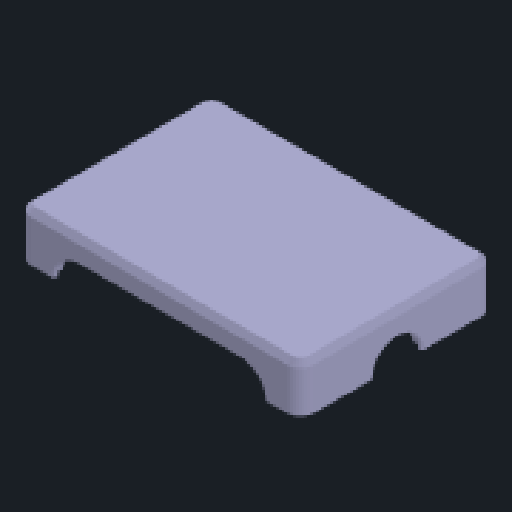
# Autodesk Inventor part: case2
Saved by Autodesk Inventor 2026.2 (Build 302298000, 298)
## iProperties
Created: 2025-10-05
Part Number: case2
Material: Generic
Document SubType Name: Modeling
Designer: micyg
Density: 1 g/cm^3
Appearance: Default
Sheet Metal Rule: Default
Author: micyg
## iProperties of the stored document case2_3DPrint.ipt
Created: 2025-10-05
Part Number: case2_3DPrint
Material: Generic
Document SubType Name: Modeling
Designer: micyg
Density: 1 g/cm^3
Appearance: Default
Author: micyg
Autodesk Inventor part; units mm, degrees
ref_plane "YZ Plane" through (0, 0, 0) normal (1, 0, 0) x (0, 1, 0)
ref_plane "XZ Plane" through (0, 0, 0) normal (0, 1, 0) x (-1, 0, 0)
ref_plane "XY Plane" through (0, 0, 0) normal (0, 0, 1) x (1, 0, 0)
sketch "Sketch1" plane through (0, 0, 0) normal (0, 1, 0) x (-1, 0, 0)
  line L0 (0, 0) -> (105, 0)
  line L1 (105, 0) -> (105, -72)
  line L2 (105, -72) -> (0, -72)
  line L3 (0, -72) -> (0, 0)
  dimension "d0" = 105
  dimension "d1" = 72
  constraints: 8 end point, 2 parallel, 1 horizontal, 1 perpendicular
  measures "d0" distance of L1.end L2.end
  measures "d1" distance of L0.end L1.end
extrude "Extrusion1" add sketch "Sketch1" along normal blind 17.5
fillet "Fillet1" radius 5 4 edges at (-105, 8.75, 0) (0, 8.75, 0) (-105, 8.75, -72) (0, 8.75, -72)
chamfer "Chamfer1" distance 2 angle 45 8 edges at (-52.5, 17.5, 0) (-1.4645, 17.5, -1.4645) (0, 17.5, -36) (-1.4645, 17.5, -70.5355) (-52.5, 17.5, -72) (-103.5355, 17.5, -70.5355) (-105, 17.5, -36) (-103.5355, 17.5, -1.4645)
shell "Shell2" thickness 3 removed faces 1 at (-36.6667, 0, -24)
ref_plane "Work Plane2" through (-52.5, 0, 0) normal (1, 0, 0) x (0, 1, 0)
ref_plane "Work Plane3" through (0, 0, -36) normal (0, 0, -1) x (-1, 0, 0)
ref_plane "Work Plane4" through (0, 1.915, 0) normal (0, -1, 0) x (1, 0, 0)
sketch "Sketch19" plane through (-52.5, 0, 0) normal (1, 0, 0) x (0, 1, 0)
  line L0 (0, -3) -> (14.2574, -3) projected
  line L1 (14.2574, -3) -> (0, -3) projected
  line L2 (14.5, -5.7) -> (8.5, -5.7)
  line L3 (7.5, -5.7) -> (8.5, -6.7) construction
  line L4 (8.5, -6.7) -> (8.5, -5.7)
  line L5 (8.5, -5.7) -> (7.5, -5.7) construction
  line L6 (8.5, -6.7) -> (14.5, -12.7)
  line L7 (0, -67) -> (0, -72) projected
  line L8 (0, -5) -> (0, -67) projected
  line L9 (0, 0) -> (0, -5) projected
  line L10 (0, -5) -> (0, 0) projected
  line L11 (0, -67) -> (0, -5) projected
  line L12 (0, -72) -> (0, -67) projected
  line L13 (14.5, -3.2426) -> (14.5, -5) projected
  line L14 (14.5, -5) -> (14.5, -67) projected
  line L15 (14.5, -67) -> (14.5, -68.7574) projected
  line L16 (14.5, -68.7574) -> (14.5, -67) projected
  line L17 (14.5, -67) -> (14.5, -5) projected
  line L18 (14.5, -5) -> (14.5, -3.2426) projected
  dimension "d104" = 2.7
  dimension "d105" = 1
  dimension "d157" = 45
  dimension "d179" = 6
  constraints: 10 end point, 2 perpendicular, 2 point on line, 1 collinear
  measures "d104" distance between parallel lines of L0 L2
  measures "d105" distance from line of L3.end L2
  measures "d157" angle of L17 L6
  measures "d179" distance between parallel lines of L17 L4
extrude "Extrusion15" add sketch "Sketch19" against normal up to surface (49.5 mm away)
mirror "Mirror9" about plane through (-52.5, 0, 0) normal (1, 0, 0) of "Extrusion15"
mirror "Mirror10" about plane through (0, 0, -36) normal (0, 0, -1) of "Extrusion15", "Mirror9"
sketch "Sketch9" plane through (0, 1.915, 0) normal (0, -1, 0) x (1, 0, 0)
  arc A0 (-5, -72) -> (0, -67) centre (-5, -67) ccw projected
  line L0 (0, -5) -> (0, -67) projected
  arc A1 (0, -5) -> (-5, 0) centre (-5, -5) ccw projected
  line L1 (-100, 0) -> (-5, 0) projected
  arc A2 (-100, 0) -> (-105, -5) centre (-100, -5) ccw projected
  line L2 (-105, -67) -> (-105, -5) projected
  arc A3 (-105, -67) -> (-100, -72) centre (-100, -67) ccw projected
  line L3 (-5, -72) -> (-100, -72) projected
  line L4 (-96.5, -8.5) -> (-8.5, -8.5) construction
  line L5 (-8.5, -8.5) -> (-8.5, -63.5) construction
  line L6 (-8.5, -63.5) -> (-96.5, -63.5) construction
  line L7 (-96.5, -63.5) -> (-96.5, -8.5) construction
  circle A4 centre (-96.5, -8.5) radius 1.5
  circle A5 centre (-8.5, -8.5) radius 1.5
  circle A6 centre (-96.5, -63.5) radius 1.5
  circle A7 centre (-8.5, -63.5) radius 1.5
  line L8 (-52.5, -8.5) -> (-52.5, -63.5) construction
  line L9 (-101.5, -3.5) -> (-3.5, -3.5) construction
  line L10 (-3.5, -3.5) -> (-3.5, -68.5) construction
  line L11 (-3.5, -68.5) -> (-101.5, -68.5) construction
  line L12 (-101.5, -68.5) -> (-101.5, -3.5) construction
  line L13 (-101.5, -36) -> (-3.5, -36) construction
  line L14 (-52.5, 0) -> (-52.5, -72) construction
  line L15 (-105, -36) -> (0, -36) construction
  line L16 (-93, -3) -> (-93, -8.5)
  line L17 (-102.2, -12) -> (-102.2, -5)
  arc A8 (-96.5, -12) -> (-93, -8.5) centre (-96.5, -8.5) ccw
  line L18 (-96.5, -12) -> (-102.2, -12)
  line L19 (-100.2, -3) -> (-93, -3)
  line L20 (-93, -69) -> (-93, -63.5)
  arc A9 (-93, -63.5) -> (-96.5, -60) centre (-96.5, -63.5) ccw
  line L21 (-96.5, -60) -> (-102.2, -60)
  arc A10 (-12, -8.5) -> (-8.5, -12) centre (-8.5, -8.5) ccw
  line L22 (-3, -12) -> (-3, -5)
  line L23 (-12, -3) -> (-12, -8.5)
  line L24 (-8.5, -12) -> (-3, -12)
  line L25 (-5, -3) -> (-12, -3)
  arc A11 (-8.5, -60) -> (-12, -63.5) centre (-8.5, -63.5) ccw
  line L26 (-12, -69) -> (-12, -63.5)
  line L27 (-8.5, -60) -> (-3, -60)
  line L28 (-93, -3) -> (-95, -3)
  line L29 (-95, -3) -> (-95, -5.7)
  line L30 (-95, -5.7) -> (-93, -5.7)
  line L31 (-93, -5.7) -> (-93, -3)
  line L32 (-12, -3) -> (-10, -3)
  line L33 (-10, -3) -> (-10, -5.7)
  line L34 (-10, -5.7) -> (-12, -5.7)
  line L35 (-12, -5.7) -> (-12, -3)
  line L36 (-95, -69) -> (-95, -66.3)
  line L37 (-95, -66.3) -> (-93, -66.3)
  line L38 (-10, -69) -> (-10, -66.3)
  line L39 (-10, -66.3) -> (-12, -66.3)
  arc A12 (-3, -5) -> (-5, -3) centre (-5, -5) ccw projected
  line L40 (-5, -3) -> (-100, -3) projected
  line L41 (-3, -67) -> (-3, -5) projected
  arc A13 (0, -5) -> (-5, 0) centre (-5, -5) ccw projected
  line L42 (0, -5) -> (0, -67) projected
  line L43 (-100, 0) -> (-5, 0) projected
  arc A14 (-3, -5) -> (-5, -3) centre (-5, -5) ccw projected
  line L44 (-5, -3) -> (-100, -3) projected
  line L45 (-3, -67) -> (-3, -5) projected
  arc A15 (0, -5) -> (-5, 0) centre (-5, -5) ccw projected
  line L46 (0, -5) -> (0, -67) projected
  line L47 (-100, 0) -> (-5, 0) projected
  arc A16 (-5, -69) -> (-3, -67) centre (-5, -67) ccw projected
  line L48 (-5, -69) -> (-100, -69) projected
  arc A17 (-102, -67) -> (-100, -69) centre (-100, -67) ccw projected
  line L49 (-102, -67) -> (-102, -5) projected
  arc A18 (-100, -3) -> (-102, -5) centre (-100, -5) ccw projected
  line L50 (-100, -3) -> (-5, -3) projected
  arc A19 (-3, -5) -> (-5, -3) centre (-5, -5) ccw projected
  line L51 (-3, -5) -> (-3, -67) projected
  arc A20 (-5, -72) -> (0, -67) centre (-5, -67) ccw projected
  line L52 (0, -5) -> (0, -67) projected
  arc A21 (0, -5) -> (-5, 0) centre (-5, -5) ccw projected
  line L53 (-100, 0) -> (-5, 0) projected
  arc A22 (-100, 0) -> (-105, -5) centre (-100, -5) ccw projected
  line L54 (-105, -67) -> (-105, -5) projected
  arc A23 (-105, -67) -> (-100, -72) centre (-100, -67) ccw projected
  line L55 (-5, -72) -> (-100, -72) projected
  line L56 (-102, -6.7) -> (-102, -5.7) projected
  line L57 (-3, -6.7) -> (-102, -6.7) construction
  line L58 (-3, -5.7) -> (-3, -6.7) projected
  line L59 (-102, -5.7) -> (-3, -5.7) construction
  line L60 (-102, -66.3) -> (-102, -65.3) projected
  line L61 (-3, -66.3) -> (-102, -66.3) construction
  line L62 (-3, -65.3) -> (-3, -66.3) projected
  line L63 (-102, -65.3) -> (-3, -65.3) construction
  arc A24 (-5, -69) -> (-3, -67) centre (-5, -67) ccw projected
  arc A25 (-100, -3) -> (-102, -5) centre (-100, -5) ccw projected
  line L64 (-102, -5) -> (-102, -67) projected
  arc A26 (-102, -67) -> (-100, -69) centre (-100, -67) ccw projected
  line L65 (-100, -69) -> (-5, -69) projected
  arc A27 (-5, -72) -> (0, -67) centre (-5, -67) ccw projected
  line L66 (-5, -72) -> (-100, -72) projected
  arc A28 (-105, -67) -> (-100, -72) centre (-100, -67) ccw projected
  line L67 (-105, -67) -> (-105, -5) projected
  arc A29 (-100, 0) -> (-105, -5) centre (-100, -5) ccw projected
  line L68 (-102, -5) -> (-102, -67) projected
  line L69 (-105, -67) -> (-105, -5) projected
  arc A30 (-102, -67) -> (-100, -69) centre (-100, -67) ccw projected
  line L70 (-100, -69) -> (-5, -69) projected
  line L71 (-5, -72) -> (-100, -72) projected
  arc A31 (-105, -67) -> (-100, -72) centre (-100, -67) ccw projected
  arc A32 (-5, -69) -> (-3, -67) centre (-5, -67) ccw projected
  arc A33 (-100, -3) -> (-102, -5) centre (-100, -5) ccw projected
  arc A34 (-5, -72) -> (0, -67) centre (-5, -67) ccw projected
  arc A35 (-100, 0) -> (-105, -5) centre (-100, -5) ccw projected
  point P0 (-52.5, -36)
  point P1 (-12, -66.3)
  point P2 (-93, -66.3)
  point P3 (-10, -3)
  point P4 (-102, -60)
  point P5 (-95, -69)
  point P6 (-102, -12)
  point P7 (-10, -69)
  point P8 (-3, -67)
  dimension "d137" = 88
  dimension "d138" = 55
  dimension "d139" = 3
  dimension "d140" = 3
  dimension "d141" = 3
  dimension "d142" = 3
  dimension "d143" = 98
  dimension "d144" = 65
  dimension "d147" = 2
  dimension "d148" = 2
  dimension "d150" = 2
  dimension "d192" = 0.5
  constraints: 70 end point, 16 symmetric about line, 11 midpoint, 11 parallel, 8 centre point, 8 point on circle, 7 horizontal, 6 perpendicular, 5 coincident, 4 point on line, 4 tangent, 1 collinear, 6 other
  measures "d137" distance of L4.start L4.end
  measures "d138" distance of L6.end L4.start
  measures "d139" diameter of A4
  measures "d140" diameter of A7
  measures "d141" diameter of A5
  measures "d142" diameter of A6
  measures "d143" distance of L9.start L9.end
  measures "d144" distance of L12.start L9.start
  measures "d147" radial gap between concentric circles of A4 A8
  measures "d148" radial gap between concentric circles of A10 A5
  measures "d150" distance between parallel lines of L16 L29
  measures "d192" distance between parallel lines of L49 L12
extrude "Extrusion13" add sketch "Sketch9" against normal up to surface (12.585 mm away) contours L16 A8 L18 L49 A18 L19 L29 L30 | L34 L33 L25 A12 L22 L24 A10 L23 | L21 A9 L20 L37 L36 L48 A17 L49 | L41 A16 L48 L38 L39 L26 A11 L27
ref_plane "Work Plane6" through (0, 0, -24) normal (0, 0, -1) x (-1, 0, 0)
sketch "Sketch22" plane through (0, 0, -24) normal (0, 0, -1) x (-1, 0, 0)
  line L0 (3, 2.5) -> (15, 14.5)
  line L1 (90, 14.5) -> (102.1, 2.4)
  line L2 (3, 1.915) -> (3, 13.8) projected
  line L3 (3, 1.915) -> (3, 0) projected
  line L4 (3, 0) -> (3, 1.915) projected
  line L5 (3.2426, 14.5) -> (101.7574, 14.5) projected
  line L6 (101.7574, 14.5) -> (3.2426, 14.5) projected
  line L7 (102, 14.2574) -> (101.7574, 14.5) projected
  line L8 (101.7574, 14.5) -> (102, 14.2574) projected
  line L9 (102, 1.915) -> (102, 0) projected
  line L10 (102, 0) -> (102, 1.915) projected
  line L11 (52.5, -3.5) -> (52.5, 21) projected
  line L12 (102, 13.8) -> (102, 14.2574) projected
  line L13 (102, 14.2574) -> (102, 13.8) projected
  line L14 (3.2426, 14.5) -> (3, 14.2574) projected
  line L15 (3, 14.2574) -> (3.2426, 14.5) projected
  line L16 (3, 13.8) -> (3, 14.2574) projected
  line L17 (3, 14.2574) -> (3, 13.8) projected
  line L18 (10, 14.5) -> (95, 14.5) projected
  line L19 (95, 14.5) -> (10, 14.5) projected
  line L20 (10, 14.5) -> (95, 14.5) projected
  line L21 (95, 14.5) -> (10, 14.5) projected
  line L22 (102, 1.915) -> (102, 13.8) projected
  line L23 (102, 13.8) -> (102, 1.915) projected
  line L24 (3, 13.8) -> (3, 1.915) projected
  point P0 (3, 14.2574)
  point P1 (3.2426, 14.5)
  dimension "d184" = 12
  dimension "d185" = 45
  constraints: 4 end point, 3 point on line, 1 other
  measures "d184" distance from line of L5 L0.start
  measures "d185" angle of L6 L0
extrude "Extrusion18" add sketch "Sketch22" along normal mid plane 2 contours L2 L16 L14 L5 L0
mirror "Mirror12" about plane through (0, 0, -36) normal (0, 0, -1) of "Extrusion18"
sketch "Sketch26" plane through (0, 1.915, 0) normal (0, -1, 0) x (1, 0, 0)
  line L0 (-3, -60) -> (-3, -12) projected
  line L1 (0, -5) -> (0, -67) projected
  arc A0 (-5, -72) -> (0, -67) centre (-5, -67) ccw projected
  line L2 (-5, -72) -> (-100, -72) projected
  line L3 (-10, -5.7) -> (-10, -3) projected
  arc A1 (-3, -5) -> (-5, -3) centre (-5, -5) ccw projected
  arc A2 (0, -5) -> (-5, 0) centre (-5, -5) ccw projected
  line L4 (-100, 0) -> (-5, 0) projected
  line L5 (-10, -3) -> (-95, -3) projected
  line L6 (-12, -5.7) -> (-10, -5.7) projected
  line L7 (-12, -8.5) -> (-12, -5.7) projected
  arc A3 (-12, -8.5) -> (-8.5, -12) centre (-8.5, -8.5) ccw projected
  line L8 (-3, -12) -> (-8.5, -12) projected
  arc A4 (-100, 0) -> (-105, -5) centre (-100, -5) ccw projected
  line L9 (-105, -67) -> (-105, -5) projected
  arc A5 (-105, -67) -> (-100, -72) centre (-100, -67) ccw projected
  circle A6 centre (-96.5, -63.5) radius 1.5 projected
  circle A7 centre (-96.5, -8.5) radius 1.5 projected
  circle A8 centre (-8.5, -8.5) radius 1.5 projected
  circle A9 centre (-8.5, -63.5) radius 1.5 projected
  circle A10 centre (-8.5, -8.5) radius 1.5 projected
  circle A11 centre (-96.5, -63.5) radius 1.5 projected
  circle A12 centre (-8.5, -63.5) radius 1.5 projected
  circle A13 centre (-96.5, -8.5) radius 1.5 projected
  line L10 (-93, -5.7) -> (-93, -8.5) projected
  arc A14 (-96.5, -12) -> (-93, -8.5) centre (-96.5, -8.5) ccw projected
  line L11 (-96.5, -12) -> (-102, -12) projected
  line L12 (-102, -12) -> (-102, -5) projected
  line L13 (-100, -3) -> (-95, -3) projected
  line L14 (-95, -3) -> (-95, -5.7) projected
  line L15 (-95, -5.7) -> (-93, -5.7) projected
  line L16 (-102, -12) -> (-102, -60) projected
  line L17 (-102, -67) -> (-102, -60) projected
  line L18 (-95, -69) -> (-100, -69) projected
  line L19 (-95, -66.3) -> (-95, -69) projected
  line L20 (-93, -66.3) -> (-95, -66.3) projected
  line L21 (-93, -63.5) -> (-93, -66.3) projected
  arc A15 (-93, -63.5) -> (-96.5, -60) centre (-96.5, -63.5) ccw projected
  line L22 (-102, -60) -> (-96.5, -60) projected
  line L23 (-8.5, -60) -> (-3, -60) projected
  arc A16 (-8.5, -60) -> (-12, -63.5) centre (-8.5, -63.5) ccw projected
  line L24 (-12, -66.3) -> (-12, -63.5) projected
  line L25 (-10, -66.3) -> (-12, -66.3) projected
  line L26 (-10, -69) -> (-10, -66.3) projected
  line L27 (-95, -69) -> (-10, -69) projected
  line L28 (-10, -3) -> (-5, -3) projected
  line L29 (-3, -12) -> (-3, -5) projected
  line L30 (-3, -67) -> (-3, -60) projected
  line L31 (-5, -69) -> (-10, -69) projected
  arc A17 (-102, -67) -> (-100, -69) centre (-100, -67) ccw projected
  arc A18 (-5, -69) -> (-3, -67) centre (-5, -67) ccw projected
  arc A19 (-100, -3) -> (-102, -5) centre (-100, -5) ccw projected
  point P0 (0, 0)
extrude "Extrusion21" cut sketch "Sketch26" against normal up to surface (12.585 mm away) contours A6 | A7 | A8 | A9
sketch "Sketch30" plane through (0, 0, -5) normal (1, 0, 0) x (0, 0, -1)
  line L0 (0, 15.5) -> (62, 15.5) construction
  line L1 (0, 0) -> (0, 15.5) construction
  line L2 (0, 0) -> (62, 0) construction
  line L3 (62, 15.5) -> (62, 0) construction
  line L4 (31, 22.8) -> (31, -14.3) construction
  circle A0 centre (31, 0) radius 9
  point P0 (-5, 0)
  dimension "d160" = 18
  constraints: 1 centre point, 1 midpoint, 1 point on line
  measures "d160" diameter of A0
extrude "Extrusion22" cut sketch "Sketch30" against normal up to surface (3 mm away)
sketch "Sketch31" plane through (-5, 0, -72) normal (0, 0, -1) x (-1, 0, 0)
  line L0 (17.5, -9) -> (47.6, -9)
  arc A0 (17.5, 9) -> (17.5, -9) centre (17.5, 0) ccw
  line L1 (54.189, 9) -> (17.5, 9)
  line L2 (77.5, -9) -> (47.6, -9)
  arc A1 (77.5, -9) -> (77.5, 9) centre (77.5, 0) ccw
  line L3 (54.189, 9) -> (77.5, 9)
  line L4 (86.5, 9) -> (8.5, 9) construction
  line L5 (8.5, 9) -> (8.5, -9) construction
  line L6 (8.5, -9) -> (86.5, -9) construction
  line L7 (86.5, -9) -> (86.5, 9) construction
  line L8 (86.5, 9) -> (8.5, -9) construction
  line L9 (8.5, 9) -> (86.5, -9) construction
  line L10 (0, 15.5) -> (95, 15.5) projected
  line L11 (0, 0) -> (0, 15.5) projected
  line L12 (0, 0) -> (95, 0) projected
  line L13 (95, 15.5) -> (95, 0) projected
  line L14 (47.5, -14.3) -> (47.5, 22.8) projected
  point P0 (47.5, 0)
  point P1 (47.5, 0)
  point P2 (47.5, 0)
  point P3 (47.5, 0)
  dimension "d163" = 9
  dimension "d164" = 78
  constraints: 20 end point, 6 tangent, 5 midpoint, 4 point on circle, 3 collinear, 3 parallel, 3 point on line, 2 centre point, 1 coincident, 1 horizontal, 1 perpendicular, 1 other
  measures "d163" radius of A0
  measures "d164" distance between parallel lines of L5 L7
extrude "Extrusion23" cut sketch "Sketch31" against normal up to surface (3 mm away) contours A0 L12 L14 L0 | L14 L12 A1 L2 L0 | A0 L1 L14 L12 | L14 L1 L3 A1 L12
mirror "Mirror13" about plane through (0, 0, -36) normal (0, 0, -1) of "Extrusion23"
sketch "Sketch33" plane through (0, 0, 0) normal (0, -1, 0) x (1, 0, 0)
  line L0 (-91.5, -3) -> (-91.5, 0) projected
  line L1 (-100, 0) -> (-91.5, 0) projected
  arc A0 (-100, 0) -> (-105, -5) centre (-100, -5) ccw projected
  line L2 (-105, -67) -> (-105, -5) projected
  arc A1 (-105, -67) -> (-100, -72) centre (-100, -67) ccw projected
  line L3 (-91.5, -72) -> (-100, -72) projected
  line L4 (-91.5, -72) -> (-91.5, -69) projected
  line L5 (-91.5, -69) -> (-100, -69) projected
  arc A2 (-102, -67) -> (-100, -69) centre (-100, -67) ccw projected
  line L6 (-102, -67) -> (-102, -5) projected
  arc A3 (-100, -3) -> (-102, -5) centre (-100, -5) ccw projected
  line L7 (-100, -3) -> (-91.5, -3) projected
  line L8 (-13.5, 0) -> (-13.5, -3) projected
  line L9 (-13.5, -3) -> (-5, -3) projected
  arc A4 (-3, -5) -> (-5, -3) centre (-5, -5) ccw projected
  line L10 (-3, -5) -> (-3, -27) projected
  line L11 (-3, -27) -> (0, -27) projected
  line L12 (0, -5) -> (0, -27) projected
  arc A5 (0, -5) -> (-5, 0) centre (-5, -5) ccw projected
  line L13 (-13.5, 0) -> (-5, 0) projected
  line L14 (-13.5, -69) -> (-13.5, -72) projected
  line L15 (-5, -72) -> (-13.5, -72) projected
  arc A6 (-5, -72) -> (0, -67) centre (-5, -67) ccw projected
  line L16 (0, -45) -> (0, -67) projected
  line L17 (0, -45) -> (-3, -45) projected
  line L18 (-3, -45) -> (-3, -67) projected
  arc A7 (-5, -69) -> (-3, -67) centre (-5, -67) ccw projected
  line L19 (-5, -69) -> (-13.5, -69) projected
  arc A8 (-5, -70.6) -> (-1.4, -67) centre (-5, -67) ccw
  line L20 (-5, -70.6) -> (-13.5, -70.6)
  line L21 (-1.4, -45) -> (-1.4, -67)
  line L22 (-13.5, -1.4) -> (-5, -1.4)
  arc A9 (-1.4, -5) -> (-5, -1.4) centre (-5, -5) ccw
  line L23 (-1.4, -5) -> (-1.4, -27)
  line L24 (-103.6, -5) -> (-103.6, -67)
  arc A10 (-103.6, -67) -> (-100, -70.6) centre (-100, -67) ccw
  line L25 (-100, -70.6) -> (-91.5, -70.6)
  line L26 (-91.5, -1.4) -> (-100, -1.4)
  arc A11 (-100, -1.4) -> (-103.6, -5) centre (-100, -5) ccw
  line L27 (-13.5, 0) -> (-13.5, -3) projected
  line L28 (-91.5, -72) -> (-91.5, -69) projected
  line L29 (-91.5, -3) -> (-91.5, 0) projected
  line L30 (-3, -45) -> (-3, -27) projected
  line L31 (-1.4, -45) -> (-3, -45)
  line L32 (-3, -45) -> (-3, -27)
  line L33 (-3, -27) -> (-1.4, -27)
  line L34 (-1.4, -27) -> (-1.4, -45)
  line L35 (-91.5, -1.4) -> (-13.5, -1.4)
  line L36 (-13.5, -1.4) -> (-13.5, -3)
  line L37 (-13.5, -3) -> (-91.5, -3)
  line L38 (-91.5, -3) -> (-91.5, -1.4)
  line L39 (-5, -69) -> (-13.5, -69) projected
  line L40 (-13.5, -69) -> (-91.5, -69)
  line L41 (-91.5, -69) -> (-91.5, -70.6)
  line L42 (-91.5, -70.6) -> (-13.5, -70.6)
  line L43 (-13.5, -70.6) -> (-13.5, -69)
  point P0 (0, 0)
  point P1 (-13.5, -70.6)
  point P2 (-13.5, -1.4)
  point P3 (-91.5, -1.4)
  dimension "d174" = 1.4
  dimension "d175" = 1.4
  dimension "d176" = 1.4
  constraints: 38 end point, 8 point on circle, 6 parallel, 6 point on line, 4 centre point, 3 horizontal, 3 perpendicular, 2 tangent, 6 other
  measures "d174" distance between parallel lines of L1 L26
  measures "d175" distance between parallel lines of L13 L22
  measures "d176" distance between parallel lines of L16 L21
extrude "Extrusion25" cut sketch "Sketch33" against normal blind 1.6 contours L7 A3 L6 A2 L5 L4 L25 A10 L24 A11 L26 L0 | L0 L35 L8 L37 | L8 L22 A9 L23 L11 L10 A4 L9 | L11 L34 L17 L30 | L40 L14 L42 L4 | L17 L21 A8 L20 L14 L19 A7 L18
sketch "Sketch34" plane through (0, 0, -25) normal (0, 0, -1) x (-1, 0, 0)
  line L0 (3, 14.2574) -> (3, 2.5) projected
  line L1 (3.2426, 14.5) -> (3, 14.2574) projected
  line L2 (15, 14.5) -> (3.2426, 14.5) projected
  line L3 (15, 14.5) -> (3, 2.5) construction
  line L4 (15, 14.5) -> (3.2426, 14.5) projected
  line L5 (3.2426, 14.5) -> (15, 14.5) projected
  line L6 (101.7574, 14.5) -> (3.2426, 14.5) projected
  line L7 (3.2426, 14.5) -> (15, 14.5) projected
  line L8 (15, 14.5) -> (3.2426, 14.5) projected
  line L9 (3.2426, 14.5) -> (101.7574, 14.5) projected
  line L10 (5.6, 14.5) -> (5.6, 8.5)
  line L11 (5.6, 7.5) -> (6.6, 8.5) construction
  line L12 (5.6, 8.5) -> (6.6, 8.5)
  line L13 (6.6, 8.5) -> (12.6, 14.5)
  line L14 (5.6, 8.5) -> (5.6, 7.5) construction
  line L15 (93, 8.5) -> (12, 8.5) projected
  line L16 (12, 8.5) -> (93, 8.5) projected
  point P0 (0, 0)
  point P1 (12.6, 14.5)
  dimension "d180" = 1
  dimension "d181" = 45
  dimension "d183" = 2.6
  constraints: 10 end point, 2 collinear, 2 point on line, 2 vertical, 1 horizontal
  measures "d180" distance from line of L11.end L10
  measures "d181" angle of L9 L13
  measures "d183" distance between parallel lines of L0 L10
extrude "Extrusion26" add sketch "Sketch34" along normal up to surface (22 mm away)
chamfer "Chamfer2" distance 0.5 angle 45 7 edges at (-16.136, 6.364, 0) (-52.5, 9, 0) (-88.864, 6.364, 0) (-16.136, 6.364, -72) (-52.5, 9, -72) (-88.864, 6.364, -72) (0, 9, -36)
equation "\"BendRadius\" = Thickness"
equation "\"BendReliefWidth\" = Thickness"
equation "\"BendReliefDepth\" = 0.5 * Thickness"
equation "\"CornerReliefSize\" = 4 * Thickness"
equation "\"MinimumRemnant\" = 2 * Thickness"
equation "\"TransitionRadius\" = BendRadius"
equation "\"JacobiRadiusSize\" = BendRadius"
equation "\"GapSize\" = Thickness"
equation "\"Thickness\" = 3.048"
body "Solid1"
